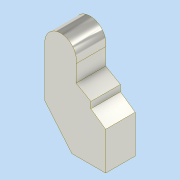
# Autodesk Inventor part: McCrea_velky_krk_walle
Saved by Autodesk Inventor 2021 (Build 250183000, 183)
## iProperties
Created: 2022-01-10
Part Number: McCrea_velky_krk_walle
Material: Generic
Document SubType Name: Modeling
Designer: student
Density: 1 g/cm^3
Appearance: Silver
Author: student
Autodesk Inventor part; units mm, degrees
ref_plane "YZ Plane" through (0, 0, 0) normal (1, 0, 0) x (0, 1, 0)
ref_plane "XZ Plane" through (0, 0, 0) normal (0, 1, 0) x (-1, 0, 0)
ref_plane "XY Plane" through (0, 0, 0) normal (0, 0, 1) x (1, 0, 0)
sketch "Sketch1" plane through (0, 0, 0) normal (0, 0, 1) x (1, 0, 0)
  line L0 (-19.9931, 0) -> (-11.9931, 0)
  line L1 (-11.9931, 0) -> (-11.9931, 9)
  line L2 (-19.9931, 0) -> (-26.421, 7.6604)
  line L3 (-26.421, 7.6604) -> (-26.421, 19.6604)
  line L4 (-11.9931, 9) -> (-15.4931, 11.4507)
  line L5 (-15.4931, 11.4507) -> (-15.4931, 12.9507)
  line L6 (-15.4931, 12.9507) -> (-18.9931, 14.9715)
  line L7 (-18.9931, 14.9715) -> (-18.9931, 18.9715)
  arc A0 (-18.9931, 18.9715) -> (-26.421, 19.6604) centre (-22.6751, 19.6604) ccw
  line L8 (-31.7243, 0) -> (5.2874, 0) projected
  point P0 (0, 0)
  dimension "d0" = 8
  dimension "d1" = 9
  dimension "d2" = 3.5
  dimension "d4" = 3.5
  dimension "d5" = 10
  dimension "d6" = 12
  dimension "d7" = 1.5
  dimension "d9" = 130
  dimension "d10" = 125
  dimension "d12" = 4
  dimension "d13" = 120
  constraints: 16 end point, 2 point on circle, 2 vertical, 1 centre point, 1 collinear, 1 parallel, 1 perpendicular, 1 tangent
  measures "d0" distance of L0.start L0.end
  measures "d1" distance of L0.end L1.end
  measures "d2" horizontal distance of L1.end L4.end
  measures "d4" horizontal distance of L5.end L6.end
  measures "d5" distance of L0.start L2.end
  measures "d6" distance of L2.end L3.end
  measures "d7" distance of L4.end L5.end
  measures "d9" angle of L0 L2
  measures "d10" angle of L1 L4
  measures "d12" distance of L6.end L7.end
  measures "d13" angle of L5 L6
extrude "Extrusion1" add sketch "Sketch1" along normal blind 7
body "Solid1"
